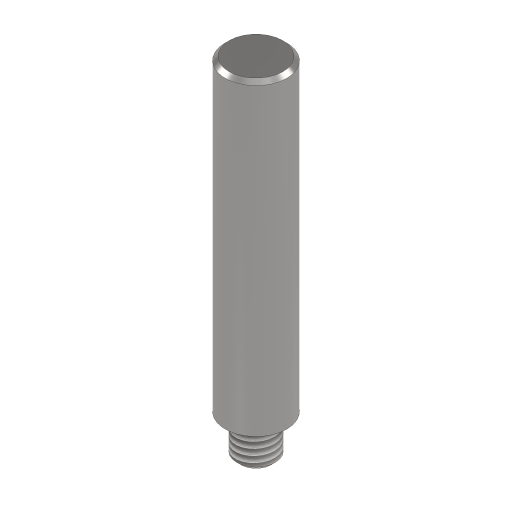
# Autodesk Inventor part: OringM5Wrench
Saved by Autodesk Inventor 2024.2 (Build 282272000, 272)
## iProperties
Created: 2022-12-02
Part Number: OringM5Wrench
Material: Stainless Steel, 440C
Document SubType Name: Modeling
Designer: kuzmin
Density: 7.75 g/cm^3
Appearance: Semi-Polished
Author: kuzmin
Autodesk Inventor part; units mm, degrees
ref_plane "YZ Plane" through (0, 0, 0) normal (1, 0, 0) x (0, 1, 0)
ref_plane "XZ Plane" through (0, 0, 0) normal (0, 1, 0) x (-1, 0, 0)
ref_plane "XY Plane" through (0, 0, 0) normal (0, 0, 1) x (1, 0, 0)
sketch "Sketch2" plane through (0, 0, 0) normal (0, 0, 1) x (1, 0, 0)
  line L0 (2.5, 0) -> (2.5, 5)
  line L1 (2.5, 5) -> (4, 5)
  line L2 (4, 5) -> (4, 45)
  line L3 (0, 0) -> (0, 45)
  line L4 (0, 0) -> (2.5, 0)
  line L5 (4, 45) -> (0, 45)
  point P0 (0, 25)
  dimension "d2" = 5
  dimension "d3" = 40
  dimension "d4" = 8
  dimension "d5" = 5
  constraints: 12 end point, 2 horizontal, 1 perpendicular, 1 point on line, 1 vertical
  measures "d2" distance of L0.start L0.end
  measures "d3" distance of L1.end L2.end
  measures "d4" diameter of L2 L3
  measures "d5" diameter of L0 L3
revolve "Revolution1" add sketch "Sketch2" angle 360 about axis through (0, 0, 0) along (0, 1, 0)
thread "Thread1" size "M5x0.8" class "6g" standard "ANSI Metric M Profile" full length
chamfer "Chamfer1" distance 0.5 angle 45 2 edges at (-4, 45, 0) (-2.5, 0, 0)
body "Solid1"
